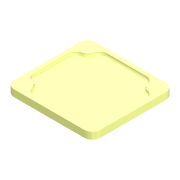
# Autodesk Inventor part: Machined Lid
Saved by Autodesk Inventor 2020.1 (Build 241239000, 239)
## iProperties
Created: 2019-10-07
Part Number: Machined Lid
Material: Aluminum 6061
Document SubType Name: Modeling
Designer: thom_tremblay
Density: 2.7 g/cm^3
Appearance: Satin - Lemon Chiffon
Author: thom_tremblay
Autodesk Inventor part; units mm, degrees
ref_plane "YZ Plane" through (0, 0, 0) normal (1, 0, 0) x (0, 1, 0)
ref_plane "XZ Plane" through (0, 0, 0) normal (0, 1, 0) x (-1, 0, 0)
ref_plane "XY Plane" through (0, 0, 0) normal (0, 0, 1) x (1, 0, 0)
sketch "Sketch1" plane through (0, 0, 0) normal (0, 1, 0) x (-1, 0, 0)
  line L0 (173.4504, -76.1021) -> (92.9116, -76.1021)
  line L1 (92.9116, -76.1021) -> (92.9116, 0)
  line L2 (92.9116, 0) -> (173.4504, 0)
  line L3 (173.4504, 0) -> (173.4504, -76.1021)
  point P0 (0, 0)
  constraints: 8 end point, 2 parallel, 1 horizontal, 1 perpendicular
extrude "Extrusion1" add sketch "Sketch1" along normal blind 6.35
fillet "Fillet1" radius 7.62 4 edges at (-173.4504, 3.175, 0) (-173.4504, 3.175, -76.1021) (-92.9116, 3.175, -76.1021) (-92.9116, 3.175, 0)
sketch "Sketch2" plane through (0, 6.35, 0) normal (0, 1, 0) x (1, 0, 0)
  arc A0 (-165.8304, 76.1021) -> (-173.4504, 68.4821) centre (-165.8304, 68.4821) ccw projected
  line L0 (-100.5316, 76.1021) -> (-165.8304, 76.1021) projected
  circle A1 centre (-165.8304, 68.4821) radius 7.62
  arc A2 (-173.4504, 7.62) -> (-165.8304, 0) centre (-165.8304, 7.62) ccw projected
  circle A3 centre (-165.8304, 7.62) radius 7.62
  arc A4 (-100.5316, 0) -> (-92.9116, 7.62) centre (-100.5316, 7.62) ccw projected
  circle A5 centre (-100.5316, 7.62) radius 7.62
  arc A6 (-92.9116, 68.4821) -> (-100.5316, 76.1021) centre (-100.5316, 68.4821) ccw projected
  circle A7 centre (-100.5316, 68.4821) radius 7.62
  line L1 (-169.6404, 72.2921) -> (-96.7216, 72.2921)
  line L2 (-96.7216, 72.2921) -> (-96.7216, 3.81)
  line L3 (-96.7216, 3.81) -> (-169.6404, 3.81)
  line L4 (-169.6404, 3.81) -> (-169.6404, 72.2921)
  line L5 (-173.4504, 68.4821) -> (-173.4504, 7.62) projected
  point P0 (0, 0)
  point P1 (-169.6404, 38.051)
  point P2 (-173.4504, 38.051)
  point P3 (-133.181, 72.2921)
  point P4 (-133.181, 76.1021)
  point P5 (-169.6404, 61.8829)
  point P6 (-169.6404, 14.2191)
  point P7 (-159.2312, 3.81)
  point P8 (-107.1307, 3.81)
  point P9 (-96.7216, 14.2191)
  point P10 (-96.7216, 61.8829)
  point P11 (-107.1307, 72.2921)
  point P12 (-159.2312, 72.2921)
  dimension "d3" = 3.81
  dimension "d4" = 3.81
  constraints: 8 end point, 4 coincident, 4 midpoint, 2 parallel, 1 horizontal, 1 horizontal alignment, 1 perpendicular, 1 vertical alignment, 12 other
  measures "d3" distance between parallel lines of L5 L4
  measures "d4" distance between parallel lines of L0 L1
extrude "Extrusion2" cut sketch "Sketch2" against normal blind 2.54 contours L1 A7 L2 A5 L3 A3 L4 A1
fillet "Fillet2" radius 7.62 8 edges at (-169.6404, 5.08, -14.2191) (-159.2312, 5.08, -3.81) (-169.6404, 5.08, -61.8829) (-159.2312, 5.08, -72.2921) (-107.1307, 5.08, -72.2921) (-96.7216, 5.08, -61.8829) (-96.7216, 5.08, -14.2191) (-107.1307, 5.08, -3.81)
fillet "Fillet3" radius 2.54 16 edges at (-155.7406, 3.81, -5.4059) (-160.4422, 3.81, -13.0082) (-168.0445, 3.81, -17.7098) (-169.6404, 3.81, -38.051) (-168.0445, 3.81, -58.3923) (-160.4422, 3.81, -63.0939) (-155.7406, 3.81, -70.6962) (-133.181, 3.81, -72.2921) (-110.6214, 3.81, -70.6962) (-105.9198, 3.81, -63.0939) (-98.3175, 3.81, -58.3923) (-96.7216, 3.81, -38.051) (-98.3175, 3.81, -17.7098) (-105.9198, 3.81, -13.0082) (-110.6214, 3.81, -5.4059) (-133.181, 3.81, -3.81)
equation "\"d4\" = d3"
body "Solid1"
